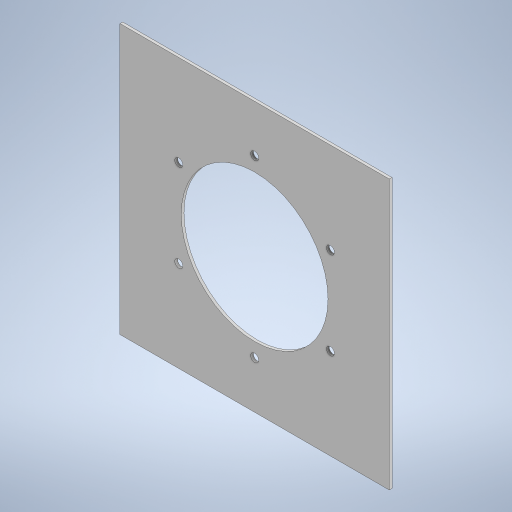
# Autodesk Inventor part: uppe sheet
Saved by Autodesk Inventor 2023 (Build 270158000, 158)
## iProperties
Created: 2023-04-27
Part Number: uppe sheet
Material: Generic
Document SubType Name: Modeling
Designer: alexa
Density: 1 g/cm^3
Appearance: Default
Author: alexa
Autodesk Inventor part; units mm, degrees
ref_plane "YZ Plane" through (0, 0, 0) normal (1, 0, 0) x (0, 1, 0)
ref_plane "XZ Plane" through (0, 0, 0) normal (0, 1, 0) x (-1, 0, 0)
ref_plane "XY Plane" through (0, 0, 0) normal (0, 0, 1) x (1, 0, 0)
sketch "Sketch1" plane through (0, 0, 0) normal (0, 0, 1) x (1, 0, 0)
  circle A0 centre (0, 0) radius 54.5
  line L0 (-100, 100) -> (100, 100)
  line L1 (100, 100) -> (100, -100)
  line L2 (100, -100) -> (-100, -100)
  line L3 (-100, -100) -> (-100, 100)
  dimension "d0" = 109
  dimension "d3" = 200
  dimension "d4" = 200
  constraints: 8 end point, 2 parallel, 1 centre point, 1 coincident, 1 horizontal, 1 perpendicular
  measures "d0" diameter of A0
  measures "d3" distance of L1.end L2.end
  measures "d4" distance of L0.end L1.end
extrude "Extrusion1" add sketch "Sketch1" along normal blind 2
sketch "Sketch2" plane through (0, 0, 2) normal (0, 0, 1) x (1, 0, 0)
  circle A0 centre (0, 65) radius 3
  circle A1 centre (-56.2917, 32.5) radius 3
  circle A2 centre (-56.2917, -32.5) radius 3
  circle A3 centre (0, -65) radius 3
  circle A4 centre (56.2917, -32.5) radius 3
  circle A5 centre (56.2917, 32.5) radius 3
  circle A6 centre (0, 0) radius 65
  dimension "d8" = 6
  dimension "d11" = 360
  constraints: 6 centre point, 1 coincident, 16 other
  measures "d8" diameter of A0
extrude "Extrusion2" cut sketch "Sketch2" against normal blind 2 contours A0 A6 | A6 A0 | A6 A1 | A1 A6 | A6 A5 | A5 A6 | A6 A2 | A2 A6 | A6 A4 | A4 A6 | A6 A3 | A3 A6
body "Solid1"
